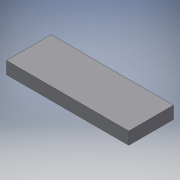
# Autodesk Inventor part: CHAPA_APOIO_SUPERIOR_EIXO_X
Saved by Autodesk Inventor 2018 (Build 220112000, 112)
## iProperties
Created: 2018-10-11
Part Number: CHAPA_APOIO_SUPERIOR_EIXO_X
Material: Genérico
Document SubType Name: Modeling
Designer: Usuario
Density: 1 g/cm^3
Appearance: Padrão
Author: Usuario
Autodesk Inventor part; units mm, degrees
ref_plane "YZ Plane" through (0, 0, 0) normal (1, 0, 0) x (0, 1, 0)
ref_plane "XZ Plane" through (0, 0, 0) normal (0, 1, 0) x (-1, 0, 0)
ref_plane "XY Plane" through (0, 0, 0) normal (0, 0, 1) x (1, 0, 0)
sketch "Esboço2" plane through (0, 0, 0) normal (0, 0, 1) x (1, 0, 0)
  line L0 (0, 12.7) -> (125, 12.7)
  line L1 (125, 12.7) -> (125, -85.3)
  line L2 (125, -85.3) -> (0, -85.3)
  line L3 (0, -85.3) -> (0, 12.7)
  dimension "d3" = 98
  dimension "d4" = 125
  constraints: 8 end point, 1 horizontal, 1 perpendicular
  measures "d3" distance of L2.end L0.start
  measures "d4" distance of L1.end L2.end
extrude "Extrusão2" add sketch "Esboço2" along normal blind 12.7
